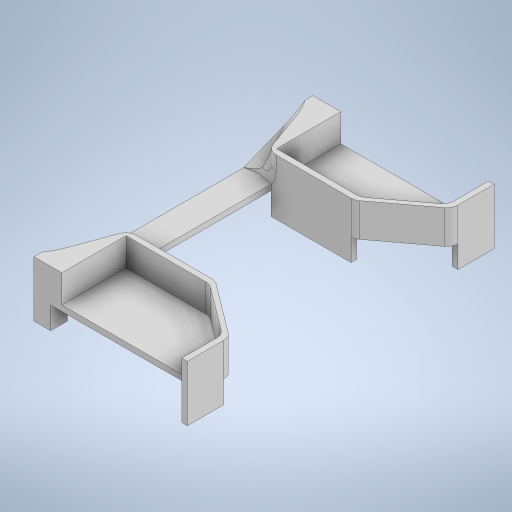
# Autodesk Inventor part: Obj2
Saved by Autodesk Inventor 2023.1 (Build 271208000, 208)
## iProperties
Created: 2023-04-24
Part Number: Obj2
Material: Generisch
Document SubType Name: Sheet Metal
Designer: marco
Density: 1 g/cm^3
Sheet Metal Rule: Standard_mm
Appearance: Vorgabe
Author: marco
Autodesk Inventor part; units mm, degrees
ref_plane "YZ Plane" through (0, 0, 0) normal (1, 0, 0) x (0, 1, 0)
ref_plane "XZ Plane" through (0, 0, 0) normal (0, 1, 0) x (-1, 0, 0)
ref_plane "XY Plane" through (0, 0, 0) normal (0, 0, 1) x (1, 0, 0)
sketch "Skizze1" plane through (0, 0, 0) normal (0, 1, 0) x (-1, 0, 0)
  line L0 (0, 0) -> (25, 0)
  line L1 (25, 0) -> (25, -25)
  line L2 (25, -25) -> (0, -25)
  line L3 (0, -25) -> (0, 0)
  line L4 (0, 0) -> (25, 0)
  line L5 (25, 0) -> (25, 15)
  line L6 (25, 15) -> (0, 15)
  line L7 (0, 15) -> (0, 0)
  line L8 (0, -25) -> (25, -25)
  line L9 (25, -25) -> (25, -40)
  line L10 (25, -40) -> (0, -40)
  line L11 (0, -40) -> (0, -25)
  line L12 (25, -40) -> (30, -40)
  line L13 (30, -40) -> (30, 15)
  line L14 (30, 15) -> (25, 15)
  line L15 (25, 15) -> (25, -40)
  line L16 (0, 15) -> (0, 7.5)
  line L17 (25, 0) -> (10, 0)
  line L18 (10, 0) -> (0, 7.5)
  line L19 (0, -40) -> (0, -32.5)
  line L20 (0, -32.5) -> (10, -25)
  line L21 (25, 0) -> (30, 0)
  line L22 (30, 0) -> (30, 5)
  line L23 (30, 5) -> (25, 0)
  line L24 (25, -25) -> (30, -30)
  line L25 (30, 15) -> (30, 5)
  line L26 (25, 0) -> (10, 0)
  line L27 (10, 0) -> (10, 1)
  line L28 (10, 1) -> (25, 1)
  line L29 (25, 1) -> (25, 0)
  line L30 (25, -25) -> (10, -25)
  line L31 (10, -25) -> (10, -26)
  line L32 (10, -26) -> (25, -26)
  line L33 (25, -26) -> (25, -25)
  line L34 (10, -26) -> (0, -33.5)
  line L35 (10, 1) -> (0, 8.5)
  line L36 (0, 7.5) -> (1, 7.5)
  line L37 (1, 7.5) -> (1, 15)
  line L38 (1, 15) -> (0, 15)
  line L39 (0, 15) -> (0, 7.5)
  line L40 (0, -40) -> (1, -40)
  line L41 (1, -40) -> (1, -32.5)
  line L42 (1, -32.5) -> (0, -32.5)
  line L43 (0, -32.5) -> (0, -40)
  point P0 (1, -32.75)
  point P1 (1, 7.75)
  dimension "d0" = 25
  dimension "d1" = 25
  dimension "d2" = 25
  dimension "d3" = 15
  dimension "d4" = 15
  dimension "d5" = 5
  dimension "d6" = 7.5
  dimension "d7" = 15
  dimension "d8" = 7.5
  dimension "d9" = 5
  dimension "d10" = 1
  dimension "d11" = 1
  dimension "d12" = 1
  constraints: 88 end point, 16 parallel, 12 point on line, 10 perpendicular, 8 horizontal, 2 midpoint, 1 collinear
  measures "d0" distance of L1.end L2.end
  measures "d1" distance of L0.end L1.end
  measures "d2" distance of L6.end L5.end
  measures "d3" distance of L5.end L4.end
  measures "d4" distance of L8.end L9.end
  measures "d5" distance of L14.end L13.end
  measures "d6" distance of L6.end L16.end
  measures "d7" distance of L4.end L17.end
  measures "d8" distance of L10.end L19.end
  measures "d9" distance of L21.end L22.end
  measures "d10" distance of L26.end L27.end
  measures "d11" distance of L31.end L30.end
  measures "d12" distance of L38.end L37.end
extrude "Extrusion1" add sketch "Skizze1" along normal blind 5 contours L27 L28 L5 L0 | L18 L36 L37 L35 L27 | L7 L35 L37 L36 | L31 L34 L41 L42 L20 | L2 L9 L32 L31 | L42 L41 L34 L11 | L7 L6 L37 L35 | L34 L41 L10 L11
sketch "Skizze2" plane through (0, 0, 0) normal (0, -1, 0) x (1, 0, 0)
  line L0 (0, -32.5) -> (0, -40) projected
  line L1 (0, -40) -> (-30, -40)
  line L2 (-30, -40) -> (-30, 15)
  line L3 (-30, 15) -> (0, 15)
  line L4 (0, 15) -> (0, -40)
  line L5 (-25, -25) -> (-10, -25) projected
  line L6 (-25, -25) -> (0, -25)
  line L7 (0, -25) -> (0, 0)
  line L8 (0, 0) -> (-25, 0)
  line L9 (-25, 0) -> (-25, -25)
  line L10 (-10, -25) -> (0, -32.5) projected
  line L11 (-10, -25) -> (0, -32.5)
  line L12 (0, 7.5) -> (-10, 0) projected
  line L13 (0, -32.5) -> (0, 7.5)
  line L14 (0, 7.5) -> (-10, 0)
  dimension "d15" = 30
  constraints: 22 end point, 6 equal length, 2 horizontal, 2 perpendicular, 1 vertical
  measures "d15" distance of L2.end L3.end
extrude "Extrusion2" add sketch "Skizze2" along normal blind 1 contours L0 L1 L2 L3 L4 L12 L8 L9 L5 L10
sketch "Skizze3" plane through (-30, 0, -40) normal (-1, 0, 0) x (0, 0, 1)
  line L0 (15, 0) -> (40, 0) projected
  line L1 (27.5, 0) -> (27.5, 6.2911)
  line L2 (15, 0) -> (15, 5) projected
  line L3 (15, 0) -> (2.5, 0)
  line L4 (55, 0) -> (0, 0) projected
  line L5 (2.5, 0) -> (2.5, 5)
  line L6 (2.5, 5) -> (15, 0)
  line L7 (40, 0) -> (52.5, 0)
  line L8 (47.75, 0) -> (55, 0) projected
  line L9 (52.5, 0) -> (52.5, 5)
  line L10 (47.75, 5) -> (55, 5) projected
  line L11 (40, 0) -> (52.5, 5)
  dimension "d19" = 12.5
  dimension "d20" = 5
  dimension "d21" = 12.5
  constraints: 14 end point, 3 perpendicular, 3 point on line, 1 midpoint
  measures "d19" distance of L0.start L3.end
  measures "d20" distance of L3.end L5.end
  measures "d21" distance of L0.end L7.end
extrude "Extrusion3" add sketch "Skizze3" against normal blind 5
sketch "Skizze4" plane through (0, 0, 0) normal (0, 1, 0) x (1, 0, 0)
  line L0 (-25, 25) -> (-30, 25) projected
  line L1 (-25, 25) -> (-25.5, 25)
  line L2 (-25, 37.5) -> (-25, 26) projected
  line L3 (-25, 25) -> (-25, 37.5)
  line L4 (-30, 37.5) -> (-25, 37.5) projected
  line L5 (-25, 37.5) -> (-30, 37.5)
  line L6 (-30, 37.5) -> (-25.5, 25)
  line L7 (-25, 25) -> (-25, 0) projected
  line L8 (-25, -1) -> (-25, -12.5) projected
  line L9 (-25, 0) -> (-25, -12.5)
  line L10 (-30, -12.5) -> (-25, -12.5) projected
  line L11 (-25, -12.5) -> (-30, -12.5)
  line L12 (-25, 0) -> (-25, -1) projected
  line L13 (-25, 0) -> (-25.5, 0)
  line L14 (-30, 0) -> (-25, 0) projected
  line L15 (-30, -12.5) -> (-25.5, 0)
  point P0 (0, 0)
  dimension "d24" = 0.5
  constraints: 16 end point, 4 collinear, 2 point on line
  measures "d24" distance of L0.start L1.end
extrude "Extrusion4" add sketch "Skizze4" along normal blind 5
sketch "Skizze5" plane through (0, 0, 0) normal (0, 1, 0) x (1, 0, 0)
  line L0 (-30, -15) -> (-30, 40) projected
  line L1 (-1, 40) -> (-1, 32.75) projected
  line L2 (-30, 40) -> (-1, 40)
  line L3 (-1, 40) -> (-1, 37.5)
  line L4 (-1, 37.5) -> (-30, 37.5)
  line L5 (-30, 37.5) -> (-30, 40)
  line L6 (-1, -15) -> (-30, -15) projected
  line L7 (-30, -15) -> (-1, -15)
  line L8 (-1, -15) -> (-1, -12.5)
  line L9 (-1, -12.5) -> (-30, -12.5)
  line L10 (-30, -12.5) -> (-30, -15)
  point P0 (0, 0)
  dimension "d27" = 2.5
  constraints: 16 end point, 4 parallel, 2 horizontal, 2 perpendicular, 2 point on line
  measures "d27" distance of L2.end L3.end
extrude "Extrusion5" cut sketch "Skizze5" against normal blind 5
fillet "Rundung1" radius 2 12 edges at (-10, 2, 0) (-10, 2, -25) (0, 2, -32.5) (0, 2, 7.5) (-1, 2.5, 7.75) (-1, 2.5, -32.75) (-10, 2.5, -26) (-10, 2.5, 1) (-27.75, 2.5, 6.25) (-25.5, 2.5, 0) (-27.75, 2.5, -31.25) (-25.5, 2.5, -25)
sketch "Skizze6" plane through (0, -1, 0) normal (0, -1, 0) x (1, 0, 0)
  line L0 (-30, -37.5) -> (-1, -37.5) projected
  line L1 (-30, -37.5) -> (-27, -37.5)
  line L2 (-27, -37.5) -> (-27, -34.5)
  line L3 (-27, -34.5) -> (-30, -34.5)
  line L4 (-30, -34.5) -> (-30, -37.5)
  line L5 (-1, 12.5) -> (-30, 12.5) projected
  line L6 (-30, 12.5) -> (-27, 12.5)
  line L7 (-27, 12.5) -> (-27, 9.5)
  line L8 (-27, 9.5) -> (-30, 9.5)
  line L9 (-30, 9.5) -> (-30, 12.5)
  line L10 (0, 15) -> (-1, 15) projected
  line L11 (0, 8.5) -> (0, 15) projected
  line L12 (-1, 15) -> (0, 15)
  line L13 (0, 15) -> (0, 8.5)
  line L14 (0, 8.5) -> (-1, 8.5)
  line L15 (-1, 8.5) -> (-1, 15)
  line L16 (0, -40) -> (-1, -40) projected
  arc A0 (-1, -33.75) -> (-1.8, -32.15) centre (-3, -33.75) ccw projected
  line L17 (0, -40) -> (-1.0157, -40)
  line L18 (-1.0157, -40) -> (-1.0157, -33.5)
  line L19 (-1.0157, -33.5) -> (0, -33.5)
  line L20 (0, -33.5) -> (0, -40)
  arc A1 (-9.4667, -26.4) -> (-10.6667, -26) centre (-10.6667, -28) ccw projected
  line L21 (-25, -25) -> (-10.6667, -25)
  line L22 (-10.6667, -25) -> (-10.6667, -26)
  line L23 (-10.6667, -26) -> (-25, -26)
  line L24 (-25, -26) -> (-25, -25)
  line L25 (-25, 0) -> (-10.6667, 0) projected
  line L26 (-25, 1) -> (-10.6667, 1) projected
  line L27 (-25, 0) -> (-10.6667, 0)
  line L28 (-10.6667, 0) -> (-10.6667, 1)
  line L29 (-10.6667, 1) -> (-25, 1)
  line L30 (-25, 1) -> (-25, 0)
  point P0 (0, 0)
  dimension "d31" = 3
  dimension "d32" = 3
  dimension "d33" = 3
  dimension "d34" = 6.5
  constraints: 48 end point, 12 parallel, 6 horizontal, 6 perpendicular, 1 point on circle, 1 point on line
  measures "d31" distance of L3.end L2.end
  measures "d32" distance of L2.end L1.end
  measures "d33" distance of L6.end L7.end
  measures "d34" distance of L17.end L18.end
extrude "Extrusion6" add sketch "Skizze6" along normal blind 4
equation "\"Biegeradius\" = Stärke"
equation "\"MinimalRest\" = 2 * Stärke"
equation "\"Abstandsgröße\" = Stärke"
equation "\"Übergangsradius\" = Biegeradius"
equation "\"JacobiRadiusGröße\" = Biegeradius"
equation "\"GrößeEckenfreistellung\" = 4 * Stärke"
equation "\"TiefeBiegungsfreistellung\" = 0.5 * Stärke"
equation "\"BreiteBiegungsfreistellung\" = Stärke"
equation "\"Stärke\" = 0.5"
